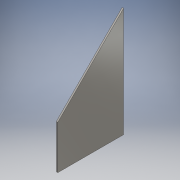
# Autodesk Inventor part: side gusset
Saved by Autodesk Inventor 2016 (Build 200138000, 138)
## iProperties
Created: 2019-03-25
Part Number: side gusset
Material: Stainless Steel, Austenitic
Document SubType Name: Modeling
Designer: benja
Density: 8 g/cm^3
Appearance: Semi-Polished
Mass: 3.93819e+06 g
Surface Area: 171645 cm^2
Volume: 492273 cm^3
Author: benja
Autodesk Inventor part; units mm, degrees
ref_plane "YZ Plane" through (0, 0, 0) normal (1, 0, 0) x (0, 1, 0)
ref_plane "XZ Plane" through (0, 0, 0) normal (0, 1, 0) x (-1, 0, 0)
ref_plane "XY Plane" through (0, 0, 0) normal (0, 0, 1) x (1, 0, 0)
sketch "Sketch1" plane through (0, 0, 0) normal (1, 0, 0) x (0, 1, 0)
  line L0 (0, 0) -> (2656.64, 0)
  line L1 (2656.64, 0) -> (2656.64, -1760)
  line L2 (2656.64, -1760) -> (0, -1760)
  line L3 (0, -1760) -> (0, 0)
  line L4 (0, 0) -> (2656.64, 2656.64)
  line L5 (0, 0) -> (2156.3058, 0) construction
  line L6 (2656.64, 0) -> (2656.64, 2656.64)
  dimension "d0" = 2656.64
  dimension "d1" = 1760
  dimension "d2" = 45
  constraints: 14 end point, 2 horizontal, 2 parallel, 1 perpendicular, 1 point on line, 1 vertical
  measures "d0" distance of L1.end L2.end
  measures "d1" distance of L0.end L1.end
  measures "d2" angle of L5 L4
extrude "Extrusion1" add sketch "Sketch1" along normal blind 60
body "Solid1"
